Autodesk Fusion 360 part; units mm, degrees
(part 2 of 3)
  arc A151 (63.8462, -218.088) -> (64.9191, -217.0151) centre (64.9191, -218.088) cw
  line L279 (63.8462, -218.088) -> (63.8462, -226.6714)
  arc A152 (51.6032, -227.7443) -> (50.5303, -226.6714) centre (51.6032, -226.6714) cw
  line L280 (51.6032, -227.7443) -> (60.1866, -227.7443)
  arc A153 (61.2596, -226.6714) -> (60.1866, -227.7443) centre (60.1866, -226.6714) cw
  line L281 (61.2596, -226.6714) -> (61.2596, -218.088)
  arc A154 (60.1866, -217.0151) -> (61.2596, -218.088) centre (60.1866, -218.088) cw
  line L282 (60.1866, -217.0151) -> (51.6032, -217.0151)
  arc A155 (50.5303, -218.088) -> (51.6032, -217.0151) centre (51.6032, -218.088) cw
  line L283 (50.5303, -218.088) -> (50.5303, -226.6714)
  arc A156 (38.2293, -227.7443) -> (37.1563, -226.6714) centre (38.2293, -226.6714) cw
  line L284 (38.2293, -227.7443) -> (46.8127, -227.7443)
  arc A157 (47.8856, -226.6714) -> (46.8127, -227.7443) centre (46.8127, -226.6714) cw
  line L285 (47.8856, -226.6714) -> (47.8856, -218.088)
  arc A158 (46.8127, -217.0151) -> (47.8856, -218.088) centre (46.8127, -218.088) cw
  line L286 (46.8127, -217.0151) -> (38.2293, -217.0151)
  arc A159 (37.1563, -218.088) -> (38.2293, -217.0151) centre (38.2293, -218.088) cw
  line L287 (37.1563, -218.088) -> (37.1563, -226.6714)
  arc A160 (64.9191, -214.9497) -> (63.8462, -213.8768) centre (64.9191, -213.8768) cw
  line L288 (64.9191, -214.9497) -> (73.5025, -214.9497)
  arc A161 (74.5755, -213.8768) -> (73.5025, -214.9497) centre (73.5025, -213.8768) cw
  line L289 (74.5755, -213.8768) -> (74.5755, -205.2933)
  arc A162 (73.5025, -204.2204) -> (74.5755, -205.2933) centre (73.5025, -205.2934) cw
  line L290 (73.5025, -204.2204) -> (64.9191, -204.2204)
  arc A163 (63.8462, -205.2933) -> (64.9191, -204.2204) centre (64.9191, -205.2934) cw
  line L291 (63.8462, -205.2933) -> (63.8462, -213.8768)
  arc A164 (51.6032, -214.9497) -> (50.5303, -213.8768) centre (51.6032, -213.8768) cw
  line L292 (51.6032, -214.9497) -> (60.1866, -214.9497)
  arc A165 (61.2596, -213.8768) -> (60.1866, -214.9497) centre (60.1866, -213.8768) cw
  line L293 (61.2596, -213.8768) -> (61.2596, -205.2933)
  arc A166 (60.1866, -204.2204) -> (61.2596, -205.2933) centre (60.1866, -205.2934) cw
  line L294 (60.1866, -204.2204) -> (51.6032, -204.2204)
  arc A167 (50.5303, -205.2933) -> (51.6032, -204.2204) centre (51.6032, -205.2934) cw
  line L295 (50.5303, -205.2933) -> (50.5303, -213.8768)
  arc A168 (38.2293, -214.9497) -> (37.1563, -213.8768) centre (38.2293, -213.8768) cw
  line L296 (38.2293, -214.9497) -> (46.8127, -214.9497)
  arc A169 (47.8856, -213.8768) -> (46.8127, -214.9497) centre (46.8127, -213.8768) cw
  line L297 (47.8856, -213.8768) -> (47.8856, -205.2933)
  arc A170 (46.8127, -204.2204) -> (47.8856, -205.2933) centre (46.8127, -205.2934) cw
  line L298 (46.8127, -204.2204) -> (38.2293, -204.2204)
  arc A171 (37.1563, -205.2933) -> (38.2293, -204.2204) centre (38.2293, -205.2934) cw
  line L299 (37.1563, -205.2933) -> (37.1563, -213.8768)
  line L300 (53.9872, -39.8421) -> (53.9872, -39.7836)
  spline S12 degree 3 poles (53.9872, -39.7836) (53.9872, -38.4968) (55.0682, -37.4761) (56.4518, -37.4761) knots 0 0 0 0 1 1 1 1
  line L301 (56.4518, -37.4761) -> (133.5511, -37.4761)
  spline S13 degree 3 poles (133.5511, -37.4761) (134.8914, -37.4761) (136.0156, -38.5138) (136.0156, -39.8421) knots 0 0 0 0 1 1 1 1
  line L302 (136.0156, -39.8421) -> (136.0156, -39.9124)
  spline S14 degree 3 poles (136.0156, -39.9124) (136.0156, -41.1992) (134.9347, -42.2081) (133.5511, -42.2081) knots 0 0 0 0 1 1 1 1
  line L303 (133.5511, -42.2081) -> (56.4518, -42.2081)
  spline S15 degree 3 poles (56.4518, -42.2081) (55.1114, -42.2081) (53.9872, -41.1704) (53.9872, -39.8421) knots 0 0 0 0 1 1 1 1
  circle A172 centre (163.266, -40.5201) radius 1.3516
  circle A173 centre (26.8902, -40.575) radius 1.3516
  circle A174 centre (163.2802, -145.4039) radius 1.3516
  circle A175 centre (26.8546, -145.4321) radius 1.3516
  circle A176 centre (163.2436, -240.8365) radius 1.3516
  circle A177 centre (26.8198, -240.7999) radius 1.3516
  line L304 (146.1597, -138.0005) -> (151.9385, -138.0005)
  line L305 (152.9385, -139.0005) -> (152.9385, -146.7816)
  line L306 (151.9385, -147.7816) -> (146.1597, -147.7816)
  line L307 (145.1597, -146.7816) -> (145.1597, -139.0005)
  line L308 (146.1591, -150.9151) -> (151.9333, -150.9151)
  line L309 (152.9333, -151.9151) -> (152.9333, -159.6975)
  line L310 (151.9333, -160.6975) -> (146.1591, -160.6975)
  line L311 (145.1591, -159.6975) -> (145.1591, -151.9151)
  arc A178 (146.1597, -138.0005) -> (145.1597, -139.0005) centre (146.1597, -139.0005) ccw
  arc A179 (152.9385, -139.0005) -> (151.9385, -138.0005) centre (151.9385, -139.0005) ccw
  arc A180 (151.9385, -147.7816) -> (152.9385, -146.7816) centre (151.9385, -146.7816) ccw
  arc A181 (145.1597, -146.7816) -> (146.1597, -147.7816) centre (146.1597, -146.7816) ccw
  arc A182 (146.1591, -150.9151) -> (145.1591, -151.9151) centre (146.1591, -151.9151) ccw
  arc A183 (152.9333, -151.9151) -> (151.9333, -150.9151) centre (151.9333, -151.9151) ccw
  arc A184 (151.9333, -160.6975) -> (152.9333, -159.6975) centre (151.9333, -159.6975) ccw
  arc A185 (145.1591, -159.6975) -> (146.1591, -160.6975) centre (146.1591, -159.6975) ccw
  line L312 (22.9151, -34.1442) -> (167.1106, -34.1442)
  line L313 (168.1106, -35.1442) -> (168.1106, -260.4512)
  line L314 (167.1106, -261.4512) -> (22.9151, -261.4512)
  line L315 (21.9151, -260.4512) -> (21.9151, -35.1442)
  arc A186 (168.1106, -35.1442) -> (167.1106, -34.1442) centre (167.1106, -35.1442) ccw
  arc A187 (167.1106, -261.4512) -> (168.1106, -260.4512) centre (167.1106, -260.4512) ccw
  arc A188 (21.9151, -260.4512) -> (22.9151, -261.4512) centre (22.9151, -260.4512) ccw
  arc A189 (22.9151, -34.1442) -> (21.9151, -35.1442) centre (22.9151, -35.1442) ccw
  point P0 (164.6176, -40.5201)
  point P1 (28.2418, -40.575)
  point P2 (164.6318, -145.4039)
  point P3 (28.2062, -145.4321)
  point P4 (164.5952, -240.8365)
  point P5 (28.1714, -240.7999)
  dimension "d1" = 1
  dimension "d2" = 1
  constraint horizontal L304
  constraint vertical L305
  constraint horizontal L306
  constraint vertical L307
  constraint horizontal L308
  constraint vertical L309
  constraint horizontal L310
  constraint vertical L311
  constraint tangent L304 A178
  constraint tangent L307 A178
  constraint tangent L304 A179
  constraint tangent L305 A179
  constraint equal A178 A179
  constraint tangent L305 A180
  constraint tangent L306 A180
  constraint equal A178 A180
  constraint tangent L306 A181
  constraint tangent L307 A181
  constraint equal A178 A181
  constraint tangent L308 A182
  constraint tangent L311 A182
  constraint equal A178 A182
  constraint tangent L308 A183
  constraint tangent L309 A183
  constraint equal A178 A183
  constraint tangent L309 A184
  constraint tangent L310 A184
  constraint equal A178 A184
  constraint tangent L310 A185
  constraint tangent L311 A185
  constraint equal A178 A185
  constraint horizontal L312
  constraint vertical L313
  constraint horizontal L314
  constraint vertical L315
  constraint tangent L312 A186
  constraint tangent L313 A186
  constraint tangent L313 A187
  constraint tangent L314 A187
  constraint equal A186 A187
  constraint tangent L314 A188
  constraint tangent L315 A188
  constraint equal A186 A188
  constraint tangent L312 A189
  constraint tangent L315 A189
  constraint equal A186 A189
  measures "d1" radius of A178
  measures "d2" radius of A186
extrude "Extrude1" add sketch "Bottom" along normal blind 3
ref_plane "WorkPlane1" through (95.0128, -147.7977, 3) normal (0, 0, 1) x (1, 0, 0)
sketch "Middle" plane through (95.0128, -147.7977, 3) normal (0, 0, 1) x (1, 0, 0)
  arc A0 (-68.0338, 82.7631) -> (-69.035, 83.7643) centre (-68.0338, 83.7643) cw
  line L0 (-68.0338, 82.7631) -> (-59.5237, 82.7631)
  arc A1 (-58.5225, 83.7643) -> (-59.5237, 82.7631) centre (-59.5237, 83.7643) cw
  line L1 (-58.5225, 83.7643) -> (-58.5225, 88.4699)
  arc A2 (-59.5237, 89.4711) -> (-58.5225, 88.4699) centre (-59.5237, 88.4699) cw
  line L2 (-59.5237, 89.4711) -> (-68.0338, 89.4711)
  arc A3 (-69.035, 88.4699) -> (-68.0338, 89.4711) centre (-68.0338, 88.4699) cw
  line L3 (-69.035, 88.4699) -> (-69.035, 83.7643)
  arc A4 (-68.0338, 71.5687) -> (-69.035, 72.5699) centre (-68.0338, 72.5699) cw
  line L4 (-68.0338, 71.5687) -> (-59.5237, 71.5687)
  arc A5 (-58.5225, 72.5699) -> (-59.5237, 71.5687) centre (-59.5237, 72.5699) cw
  line L5 (-58.5225, 72.5699) -> (-58.5225, 77.2755)
  arc A6 (-59.5237, 78.2767) -> (-58.5225, 77.2755) centre (-59.5237, 77.2755) cw
  line L6 (-59.5237, 78.2767) -> (-68.0338, 78.2767)
  arc A7 (-69.035, 77.2755) -> (-68.0338, 78.2767) centre (-68.0338, 77.2755) cw
  line L7 (-69.035, 77.2755) -> (-69.035, 72.5699)
  arc A8 (-68.0338, 60.3295) -> (-69.035, 61.3307) centre (-68.0338, 61.3307) cw
  line L8 (-68.0338, 60.3295) -> (-59.5237, 60.3295)
  arc A9 (-58.5225, 61.3307) -> (-59.5237, 60.3295) centre (-59.5237, 61.3307) cw
  line L9 (-58.5225, 61.3307) -> (-58.5225, 66.0363)
  arc A10 (-59.5237, 67.0375) -> (-58.5225, 66.0363) centre (-59.5237, 66.0363) cw
  line L10 (-59.5237, 67.0375) -> (-68.0338, 67.0375)
  arc A11 (-69.035, 66.0363) -> (-68.0338, 67.0375) centre (-68.0338, 66.0363) cw
  line L11 (-69.035, 66.0363) -> (-69.035, 61.3307)
  arc A12 (-68.0338, 49.0663) -> (-69.035, 50.0675) centre (-68.0338, 50.0675) cw
  line L12 (-68.0338, 49.0663) -> (-59.5237, 49.0663)
  arc A13 (-58.5225, 50.0675) -> (-59.5237, 49.0663) centre (-59.5237, 50.0675) cw
  line L13 (-58.5225, 50.0675) -> (-58.5225, 54.7731)
  arc A14 (-59.5237, 55.7743) -> (-58.5225, 54.7731) centre (-59.5237, 54.7731) cw
  line L14 (-59.5237, 55.7743) -> (-68.0338, 55.7743)
  arc A15 (-69.035, 54.7731) -> (-68.0338, 55.7743) centre (-68.0338, 54.7731) cw
  line L15 (-69.035, 54.7731) -> (-69.035, 50.0675)
  arc A16 (-68.0338, 37.8539) -> (-69.035, 38.8551) centre (-68.0338, 38.8551) cw
  line L16 (-68.0338, 37.8539) -> (-59.5237, 37.8539)
  arc A17 (-58.5225, 38.8551) -> (-59.5237, 37.8539) centre (-59.5237, 38.8551) cw
  line L17 (-58.5225, 38.8551) -> (-58.5225, 43.5607)
  arc A18 (-59.5237, 44.5619) -> (-58.5225, 43.5607) centre (-59.5237, 43.5607) cw
  line L18 (-59.5237, 44.5619) -> (-68.0338, 44.5619)
  arc A19 (-69.035, 43.5607) -> (-68.0338, 44.5619) centre (-68.0338, 43.5607) cw
  line L19 (-69.035, 43.5607) -> (-69.035, 38.8551)
  arc A20 (-68.0338, 26.6171) -> (-69.035, 27.6183) centre (-68.0338, 27.6183) cw
  line L20 (-68.0338, 26.6171) -> (-59.5237, 26.6171)
  arc A21 (-58.5225, 27.6183) -> (-59.5237, 26.6171) centre (-59.5237, 27.6183) cw
  line L21 (-58.5225, 27.6183) -> (-58.5225, 32.3239)
  arc A22 (-59.5237, 33.3251) -> (-58.5225, 32.3239) centre (-59.5237, 32.3239) cw
  line L22 (-59.5237, 33.3251) -> (-68.0338, 33.3251)
  arc A23 (-69.035, 32.3239) -> (-68.0338, 33.3251) centre (-68.0338, 32.3239) cw
  line L23 (-69.035, 32.3239) -> (-69.035, 27.6183)
  arc A24 (59.9614, 26.5376) -> (58.9602, 27.5388) centre (59.9614, 27.5388) cw
  line L24 (59.9614, 26.5376) -> (68.4716, 26.5376)
  arc A25 (69.4728, 27.5388) -> (68.4716, 26.5376) centre (68.4716, 27.5388) cw
  line L25 (69.4728, 27.5388) -> (69.4728, 32.2444)
  arc A26 (68.4716, 33.2456) -> (69.4728, 32.2444) centre (68.4716, 32.2444) cw
  line L26 (68.4716, 33.2456) -> (59.9614, 33.2456)
  arc A27 (58.9602, 32.2444) -> (59.9614, 33.2456) centre (59.9614, 32.2444) cw
  line L27 (58.9602, 32.2444) -> (58.9602, 27.5388)
  arc A28 (59.9614, 37.7744) -> (58.9602, 38.7756) centre (59.9614, 38.7756) cw
  line L28 (59.9614, 37.7744) -> (68.4716, 37.7744)
  arc A29 (69.4728, 38.7756) -> (68.4716, 37.7744) centre (68.4716, 38.7756) cw
  line L29 (69.4728, 38.7756) -> (69.4728, 43.4812)
  arc A30 (68.4716, 44.4824) -> (69.4728, 43.4812) centre (68.4716, 43.4812) cw
  line L30 (68.4716, 44.4824) -> (59.9614, 44.4824)
  arc A31 (58.9602, 43.4812) -> (59.9614, 44.4824) centre (59.9614, 43.4812) cw
  line L31 (58.9602, 43.4812) -> (58.9602, 38.7756)
  arc A32 (59.9614, 49.0133) -> (58.9602, 50.0145) centre (59.9614, 50.0145) cw
  line L32 (59.9614, 49.0133) -> (68.4716, 49.0133)
  arc A33 (69.4728, 50.0145) -> (68.4716, 49.0133) centre (68.4716, 50.0145) cw
  line L33 (69.4728, 50.0145) -> (69.4728, 54.7201)
  arc A34 (68.4716, 55.7213) -> (69.4728, 54.7201) centre (68.4716, 54.7201) cw
  line L34 (68.4716, 55.7213) -> (59.9614, 55.7213)
  arc A35 (58.9602, 54.7201) -> (59.9614, 55.7213) centre (59.9614, 54.7201) cw
  line L35 (58.9602, 54.7201) -> (58.9602, 50.0145)
  arc A36 (59.9614, 60.2236) -> (58.9602, 61.2248) centre (59.9614, 61.2248) cw
  line L36 (59.9614, 60.2236) -> (68.4716, 60.2236)
  arc A37 (69.4728, 61.2248) -> (68.4716, 60.2236) centre (68.4716, 61.2248) cw
  line L37 (69.4728, 61.2248) -> (69.4728, 65.9304)
  arc A38 (68.4716, 66.9316) -> (69.4728, 65.9304) centre (68.4716, 65.9304) cw
  line L38 (68.4716, 66.9316) -> (59.9614, 66.9316)
  arc A39 (58.9602, 65.9304) -> (59.9614, 66.9316) centre (59.9614, 65.9304) cw
  line L39 (58.9602, 65.9304) -> (58.9602, 61.2248)
  arc A40 (59.9614, 71.4892) -> (58.9602, 72.4904) centre (59.9614, 72.4904) cw
  line L40 (59.9614, 71.4892) -> (68.4716, 71.4892)
  arc A41 (69.4728, 72.4904) -> (68.4716, 71.4892) centre (68.4716, 72.4904) cw
  line L41 (69.4728, 72.4904) -> (69.4728, 77.196)
  arc A42 (68.4716, 78.1972) -> (69.4728, 77.196) centre (68.4716, 77.196) cw
  line L42 (68.4716, 78.1972) -> (59.9614, 78.1972)
  arc A43 (58.9602, 77.196) -> (59.9614, 78.1972) centre (59.9614, 77.196) cw
  line L43 (58.9602, 77.196) -> (58.9602, 72.4904)
  arc A44 (59.9614, 82.7631) -> (58.9602, 83.7643) centre (59.9614, 83.7643) cw
  line L44 (59.9614, 82.7631) -> (68.4716, 82.7631)
  arc A45 (69.4728, 83.7643) -> (68.4716, 82.7631) centre (68.4716, 83.7643) cw
  line L45 (69.4728, 83.7643) -> (69.4728, 88.4699)
  arc A46 (68.4716, 89.4711) -> (69.4728, 88.4699) centre (68.4716, 88.4699) cw
  line L46 (68.4716, 89.4711) -> (59.9614, 89.4711)
  arc A47 (58.9602, 88.4699) -> (59.9614, 89.4711) centre (59.9614, 88.4699) cw
  line L47 (58.9602, 88.4699) -> (58.9602, 83.7643)
  arc A48 (-54.8782, 0.767) -> (-55.8794, 1.7682) centre (-54.8782, 1.7682) cw
  line L48 (-54.8782, 0.767) -> (-43.6448, 0.767)
  arc A49 (-42.6436, 1.7682) -> (-43.6448, 0.767) centre (-43.6448, 1.7682) cw
  line L49 (-42.6436, 1.7682) -> (-42.6436, 7.8755)
  arc A50 (-43.6448, 8.8767) -> (-42.6436, 7.8755) centre (-43.6448, 7.8755) cw
  line L50 (-43.6448, 8.8767) -> (-54.8782, 8.8767)
  arc A51 (-55.8794, 7.8755) -> (-54.8782, 8.8767) centre (-54.8782, 7.8755) cw
  line L51 (-55.8794, 7.8755) -> (-55.8794, 1.7682)
  arc A52 (-54.8782, -12.0499) -> (-55.8794, -11.0487) centre (-54.8782, -11.0487) cw
  line L52 (-54.8782, -12.0499) -> (-43.6448, -12.0499)
  arc A53 (-42.6436, -11.0487) -> (-43.6448, -12.0499) centre (-43.6448, -11.0487) cw
  line L53 (-42.6436, -11.0487) -> (-42.6436, -4.9414)
  arc A54 (-43.6448, -3.9402) -> (-42.6436, -4.9414) centre (-43.6448, -4.9414) cw
  line L54 (-43.6448, -3.9402) -> (-54.8782, -3.9402)
  arc A55 (-55.8794, -4.9414) -> (-54.8782, -3.9402) centre (-54.8782, -4.9414) cw
  line L55 (-55.8794, -4.9414) -> (-55.8794, -11.0487)
  arc A56 (-54.8782, -25.4495) -> (-55.8794, -24.4483) centre (-54.8782, -24.4483) cw
  line L56 (-54.8782, -25.4495) -> (-43.6448, -25.4495)
  arc A57 (-42.6436, -24.4483) -> (-43.6448, -25.4495) centre (-43.6448, -24.4483) cw
  line L57 (-42.6436, -24.4483) -> (-42.6436, -18.3411)
  arc A58 (-43.6448, -17.3399) -> (-42.6436, -18.3411) centre (-43.6448, -18.3411) cw
  line L58 (-43.6448, -17.3399) -> (-54.8782, -17.3399)
  arc A59 (-55.8794, -18.3411) -> (-54.8782, -17.3399) centre (-54.8782, -18.3411) cw
  line L59 (-55.8794, -18.3411) -> (-55.8794, -24.4483)
  arc A60 (-54.8782, -38.5373) -> (-55.8794, -37.5362) centre (-54.8782, -37.5362) cw
  line L60 (-54.8782, -38.5373) -> (-43.6448, -38.5373)
  arc A61 (-42.6436, -37.5362) -> (-43.6448, -38.5373) centre (-43.6448, -37.5362) cw
  line L61 (-42.6436, -37.5362) -> (-42.6436, -31.4289)
  arc A62 (-43.6448, -30.4277) -> (-42.6436, -31.4289) centre (-43.6448, -31.4289) cw
  line L62 (-43.6448, -30.4277) -> (-54.8782, -30.4277)
  arc A63 (-55.8794, -31.4289) -> (-54.8782, -30.4277) centre (-54.8782, -31.4289) cw
  line L63 (-55.8794, -31.4289) -> (-55.8794, -37.5362)
  arc A64 (-54.8782, -51.5721) -> (-55.8794, -50.5709) centre (-54.8782, -50.5709) cw
  line L64 (-54.8782, -51.5721) -> (-43.6448, -51.5721)
  arc A65 (-42.6436, -50.5709) -> (-43.6448, -51.5721) centre (-43.6448, -50.5709) cw
  line L65 (-42.6436, -50.5709) -> (-42.6436, -44.4636)
  arc A66 (-43.6448, -43.4624) -> (-42.6436, -44.4636) centre (-43.6448, -44.4636) cw
  line L66 (-43.6448, -43.4624) -> (-54.8782, -43.4624)
  arc A67 (-55.8794, -44.4636) -> (-54.8782, -43.4624) centre (-54.8782, -44.4636) cw
  line L67 (-55.8794, -44.4636) -> (-55.8794, -50.5709)
  arc A68 (-36.9816, -51.5721) -> (-37.9828, -50.5709) centre (-36.9816, -50.5709) cw
  line L68 (-36.9816, -51.5721) -> (-25.7482, -51.5721)
  arc A69 (-24.747, -50.5709) -> (-25.7482, -51.5721) centre (-25.7482, -50.5709) cw
  line L69 (-24.747, -50.5709) -> (-24.747, -44.4636)
  arc A70 (-25.7482, -43.4624) -> (-24.747, -44.4636) centre (-25.7482, -44.4636) cw
  line L70 (-25.7482, -43.4624) -> (-36.9816, -43.4624)
  arc A71 (-37.9828, -44.4636) -> (-36.9816, -43.4624) centre (-36.9816, -44.4636) cw
  line L71 (-37.9828, -44.4636) -> (-37.9828, -50.5709)
  arc A72 (-36.9816, -38.5373) -> (-37.9828, -37.5362) centre (-36.9816, -37.5362) cw
  line L72 (-36.9816, -38.5373) -> (-25.7482, -38.5373)
  arc A73 (-24.747, -37.5362) -> (-25.7482, -38.5373) centre (-25.7482, -37.5362) cw
  line L73 (-24.747, -37.5362) -> (-24.747, -31.4289)
  arc A74 (-25.7482, -30.4277) -> (-24.747, -31.4289) centre (-25.7482, -31.4289) cw
  line L74 (-25.7482, -30.4277) -> (-36.9816, -30.4277)
  arc A75 (-37.9828, -31.4289) -> (-36.9816, -30.4277) centre (-36.9816, -31.4289) cw
  line L75 (-37.9828, -31.4289) -> (-37.9828, -37.5362)
  arc A76 (-36.9816, -25.4495) -> (-37.9828, -24.4483) centre (-36.9816, -24.4483) cw
  line L76 (-36.9816, -25.4495) -> (-25.7482, -25.4495)
  arc A77 (-24.747, -24.4483) -> (-25.7482, -25.4495) centre (-25.7482, -24.4483) cw
  line L77 (-24.747, -24.4483) -> (-24.747, -18.3411)
  arc A78 (-25.7482, -17.3399) -> (-24.747, -18.3411) centre (-25.7482, -18.3411) cw
  line L78 (-25.7482, -17.3399) -> (-36.9816, -17.3399)
  arc A79 (-37.9828, -18.3411) -> (-36.9816, -17.3399) centre (-36.9816, -18.3411) cw
  line L79 (-37.9828, -18.3411) -> (-37.9828, -24.4483)
  arc A80 (-36.9816, -12.0499) -> (-37.9828, -11.0487) centre (-36.9816, -11.0487) cw
  line L80 (-36.9816, -12.0499) -> (-25.7482, -12.0499)
  arc A81 (-24.747, -11.0487) -> (-25.7482, -12.0499) centre (-25.7482, -11.0487) cw
  line L81 (-24.747, -11.0487) -> (-24.747, -4.9414)
  arc A82 (-25.7482, -3.9402) -> (-24.747, -4.9414) centre (-25.7482, -4.9414) cw
  line L82 (-25.7482, -3.9402) -> (-36.9816, -3.9402)
  arc A83 (-37.9828, -4.9414) -> (-36.9816, -3.9402) centre (-36.9816, -4.9414) cw
  line L83 (-37.9828, -4.9414) -> (-37.9828, -11.0487)
  arc A84 (-36.9816, 0.767) -> (-37.9828, 1.7682) centre (-36.9816, 1.7682) cw
  line L84 (-36.9816, 0.767) -> (-25.7482, 0.767)
  arc A85 (-24.747, 1.7682) -> (-25.7482, 0.767) centre (-25.7482, 1.7682) cw
  line L85 (-24.747, 1.7682) -> (-24.747, 7.8755)
  arc A86 (-25.7482, 8.8767) -> (-24.747, 7.8755) centre (-25.7482, 7.8755) cw
  line L86 (-25.7482, 8.8767) -> (-36.9816, 8.8767)
  arc A87 (-37.9828, 7.8755) -> (-36.9816, 8.8767) centre (-36.9816, 7.8755) cw
  line L87 (-37.9828, 7.8755) -> (-37.9828, 1.7682)
  arc A88 (-18.8211, 0.767) -> (-19.8223, 1.7682) centre (-18.8211, 1.7682) cw
  line L88 (-18.8211, 0.767) -> (-7.5877, 0.767)
  arc A89 (-6.5865, 1.7682) -> (-7.5877, 0.767) centre (-7.5877, 1.7682) cw
  line L89 (-6.5865, 1.7682) -> (-6.5865, 7.8755)
  arc A90 (-7.5877, 8.8767) -> (-6.5865, 7.8755) centre (-7.5877, 7.8755) cw
  line L90 (-7.5877, 8.8767) -> (-18.8211, 8.8767)
  arc A91 (-19.8223, 7.8755) -> (-18.8211, 8.8767) centre (-18.8211, 7.8755) cw
  line L91 (-19.8223, 7.8755) -> (-19.8223, 1.7682)
  arc A92 (-18.8211, -12.0499) -> (-19.8223, -11.0487) centre (-18.8211, -11.0487) cw
  line L92 (-18.8211, -12.0499) -> (-7.5877, -12.0499)
  arc A93 (-6.5865, -11.0487) -> (-7.5877, -12.0499) centre (-7.5877, -11.0487) cw
  line L93 (-6.5865, -11.0487) -> (-6.5865, -4.9414)
  arc A94 (-7.5877, -3.9402) -> (-6.5865, -4.9414) centre (-7.5877, -4.9414) cw
  line L94 (-7.5877, -3.9402) -> (-18.8211, -3.9402)
  arc A95 (-19.8223, -4.9414) -> (-18.8211, -3.9402) centre (-18.8211, -4.9414) cw
  line L95 (-19.8223, -4.9414) -> (-19.8223, -11.0487)
  arc A96 (-0.6342, 0.767) -> (-1.6354, 1.7682) centre (-0.6342, 1.7682) cw
  line L96 (-0.6342, 0.767) -> (10.5992, 0.767)
  arc A97 (11.6004, 1.7682) -> (10.5992, 0.767) centre (10.5992, 1.7682) cw
  line L97 (11.6004, 1.7682) -> (11.6004, 7.8755)
  arc A98 (10.5992, 8.8767) -> (11.6004, 7.8755) centre (10.5992, 7.8755) cw
  line L98 (10.5992, 8.8767) -> (-0.6342, 8.8767)
  arc A99 (-1.6354, 7.8755) -> (-0.6342, 8.8767) centre (-0.6342, 7.8755) cw
  line L99 (-1.6354, 7.8755) -> (-1.6354, 1.7682)
  arc A100 (-0.6342, -12.0499) -> (-1.6354, -11.0487) centre (-0.6342, -11.0487) cw
  line L100 (-0.6342, -12.0499) -> (10.5992, -12.0499)
  arc A101 (11.6004, -11.0487) -> (10.5992, -12.0499) centre (10.5992, -11.0487) cw
  line L101 (11.6004, -11.0487) -> (11.6004, -4.9414)
  arc A102 (10.5992, -3.9402) -> (11.6004, -4.9414) centre (10.5992, -4.9414) cw
  line L102 (10.5992, -3.9402) -> (-0.6342, -3.9402)
  arc A103 (-1.6354, -4.9414) -> (-0.6342, -3.9402) centre (-0.6342, -4.9414) cw
  line L103 (-1.6354, -4.9414) -> (-1.6354, -11.0487)
  arc A104 (17.3673, 0.767) -> (16.3662, 1.7682) centre (17.3673, 1.7682) cw
  line L104 (17.3673, 0.767) -> (28.6008, 0.767)
  arc A105 (29.602, 1.7682) -> (28.6008, 0.767) centre (28.6008, 1.7682) cw
  line L105 (29.602, 1.7682) -> (29.602, 7.8755)
  arc A106 (28.6008, 8.8767) -> (29.602, 7.8755) centre (28.6008, 7.8755) cw
  line L106 (28.6008, 8.8767) -> (17.3673, 8.8767)
  arc A107 (16.3662, 7.8755) -> (17.3673, 8.8767) centre (17.3673, 7.8755) cw
  line L107 (16.3662, 7.8755) -> (16.3662, 1.7682)
  arc A108 (17.3673, -12.0499) -> (16.3662, -11.0487) centre (17.3673, -11.0487) cw
  line L108 (17.3673, -12.0499) -> (28.6008, -12.0499)
  arc A109 (29.602, -11.0487) -> (28.6008, -12.0499) centre (28.6008, -11.0487) cw
  line L109 (29.602, -11.0487) -> (29.602, -4.9414)
  arc A110 (28.6008, -3.9402) -> (29.602, -4.9414) centre (28.6008, -4.9414) cw
  line L110 (28.6008, -3.9402) -> (17.3673, -3.9402)
  arc A111 (16.3662, -4.9414) -> (17.3673, -3.9402) centre (17.3673, -4.9414) cw
  line L111 (16.3662, -4.9414) -> (16.3662, -11.0487)
  arc A112 (35.4483, 0.767) -> (34.4471, 1.7682) centre (35.4483, 1.7682) cw
  line L112 (35.4483, 0.767) -> (46.6818, 0.767)
  arc A113 (47.6829, 1.7682) -> (46.6818, 0.767) centre (46.6817, 1.7682) cw
  line L113 (47.6829, 1.7682) -> (47.6829, 7.8755)
  arc A114 (46.6817, 8.8767) -> (47.6829, 7.8755) centre (46.6817, 7.8755) cw
  line L114 (46.6817, 8.8767) -> (35.4483, 8.8767)
  arc A115 (34.4471, 7.8755) -> (35.4483, 8.8767) centre (35.4483, 7.8755) cw
  line L115 (34.4471, 7.8755) -> (34.4471, 1.7682)
  arc A116 (35.4483, -12.0499) -> (34.4471, -11.0487) centre (35.4483, -11.0487) cw
  line L116 (35.4483, -12.0499) -> (46.6818, -12.0499)
  arc A117 (47.6829, -11.0487) -> (46.6818, -12.0499) centre (46.6817, -11.0487) cw
  line L117 (47.6829, -11.0487) -> (47.6829, -4.9414)
  arc A118 (46.6817, -3.9402) -> (47.6829, -4.9414) centre (46.6817, -4.9414) cw
  line L118 (46.6817, -3.9402) -> (35.4483, -3.9402)
  arc A119 (34.4471, -4.9414) -> (35.4483, -3.9402) centre (35.4483, -4.9414) cw
  line L119 (34.4471, -4.9414) -> (34.4471, -11.0487)
  arc A120 (31.3954, -29.6551) -> (30.3942, -28.6539) centre (31.3954, -28.6539) cw
  line L120 (31.3954, -29.6551) -> (39.405, -29.6551)
  arc A121 (40.4061, -28.6539) -> (39.405, -29.6551) centre (39.405, -28.6539) cw
  line L121 (40.4061, -28.6539) -> (40.4061, -20.6443)
  arc A122 (39.405, -19.6431) -> (40.4061, -20.6443) centre (39.405, -20.6443) cw
  line L122 (39.405, -19.6431) -> (31.3954, -19.6431)
  arc A123 (30.3942, -20.6443) -> (31.3954, -19.6431) centre (31.3954, -20.6443) cw
  line L123 (30.3942, -20.6443) -> (30.3942, -28.6539)
  arc A124 (46.3835, -29.614) -> (45.3823, -28.6128) centre (46.3835, -28.6128) cw
  line L124 (46.3835, -29.614) -> (54.3931, -29.614)
  arc A125 (55.3943, -28.6128) -> (54.3931, -29.614) centre (54.3931, -28.6128) cw
  line L125 (55.3943, -28.6128) -> (55.3943, -20.6033)
  arc A126 (54.3931, -19.6021) -> (55.3943, -20.6033) centre (54.3931, -20.6033) cw
  line L126 (54.3931, -19.6021) -> (46.3835, -19.6021)
  arc A127 (45.3823, -20.6033) -> (46.3835, -19.6021) centre (46.3835, -20.6033) cw
  line L127 (45.3823, -20.6033) -> (45.3823, -28.6128)
  arc A128 (-13.9242, -29.6551) -> (-14.9253, -28.6539) centre (-13.9242, -28.6539) cw
  line L128 (-13.9242, -29.6551) -> (-5.9146, -29.6551)
  arc A129 (-4.9134, -28.6539) -> (-5.9146, -29.6551) centre (-5.9146, -28.6539) cw
  line L129 (-4.9134, -28.6539) -> (-4.9134, -20.6443)
  arc A130 (-5.9146, -19.6431) -> (-4.9134, -20.6443) centre (-5.9146, -20.6443) cw
  line L130 (-5.9146, -19.6431) -> (-13.9242, -19.6431)
  arc A131 (-14.9253, -20.6443) -> (-13.9242, -19.6431) centre (-13.9242, -20.6443) cw
  line L131 (-14.9253, -20.6443) -> (-14.9253, -28.6539)
  arc A132 (1.1007, -29.6551) -> (0.0995, -28.6539) centre (1.1007, -28.6539) cw
  line L132 (1.1007, -29.6551) -> (9.1102, -29.6551)
  arc A133 (10.1114, -28.6539) -> (9.1102, -29.6551) centre (9.1102, -28.6539) cw
  line L133 (10.1114, -28.6539) -> (10.1114, -20.6443)
  arc A134 (9.1103, -19.6431) -> (10.1114, -20.6443) centre (9.1102, -20.6443) cw
  line L134 (9.1103, -19.6431) -> (1.1007, -19.6431)
  arc A135 (0.0995, -20.6443) -> (1.1007, -19.6431) centre (1.1007, -20.6443) cw
  line L135 (0.0995, -20.6443) -> (0.0995, -28.6539)
  arc A136 (16.2654, -29.6551) -> (15.2642, -28.6539) centre (16.2654, -28.6539) cw
  line L136 (16.2654, -29.6551) -> (24.275, -29.6551)
  arc A137 (25.2761, -28.6539) -> (24.275, -29.6551) centre (24.275, -28.6539) cw
  line L137 (25.2761, -28.6539) -> (25.2761, -20.6443)
  arc A138 (24.275, -19.6431) -> (25.2761, -20.6443) centre (24.275, -20.6443) cw
  line L138 (24.275, -19.6431) -> (16.2654, -19.6431)
  arc A139 (15.2642, -20.6443) -> (16.2654, -19.6431) centre (16.2654, -20.6443) cw
  line L139 (15.2642, -20.6443) -> (15.2642, -28.6539)
  arc A140 (46.3835, -44.5902) -> (45.3823, -43.589) centre (46.3835, -43.589) cw
  line L140 (46.3835, -44.5902) -> (54.3931, -44.5902)
  arc A141 (55.3943, -43.589) -> (54.3931, -44.5902) centre (54.3931, -43.589) cw
  line L141 (55.3943, -43.589) -> (55.3943, -35.5795)
  arc A142 (54.3931, -34.5783) -> (55.3943, -35.5795) centre (54.3931, -35.5795) cw
  line L142 (54.3931, -34.5783) -> (46.3835, -34.5783)
  arc A143 (45.3823, -35.5795) -> (46.3835, -34.5783) centre (46.3835, -35.5795) cw
  line L143 (45.3823, -35.5795) -> (45.3823, -43.589)
  arc A144 (31.3954, -44.6313) -> (30.3942, -43.6301) centre (31.3954, -43.6301) cw
  line L144 (31.3954, -44.6313) -> (39.405, -44.6313)
  arc A145 (40.4061, -43.6301) -> (39.405, -44.6313) centre (39.405, -43.6301) cw
  line L145 (40.4061, -43.6301) -> (40.4061, -35.6205)
  arc A146 (39.405, -34.6193) -> (40.4061, -35.6205) centre (39.405, -35.6205) cw
  line L146 (39.405, -34.6193) -> (31.3954, -34.6193)
  arc A147 (30.3942, -35.6205) -> (31.3954, -34.6193) centre (31.3954, -35.6205) cw
  line L147 (30.3942, -35.6205) -> (30.3942, -43.6301)
  arc A148 (16.2654, -44.6313) -> (15.2642, -43.6301) centre (16.2654, -43.6301) cw
  line L148 (16.2654, -44.6313) -> (24.275, -44.6313)
  arc A149 (25.2761, -43.6301) -> (24.275, -44.6313) centre (24.275, -43.6301) cw
  line L149 (25.2761, -43.6301) -> (25.2761, -35.6205)
  arc A150 (24.275, -34.6193) -> (25.2761, -35.6205) centre (24.275, -35.6205) cw
  line L150 (24.275, -34.6193) -> (16.2654, -34.6193)
  arc A151 (15.2642, -35.6205) -> (16.2654, -34.6193) centre (16.2654, -35.6205) cw
  line L151 (15.2642, -35.6205) -> (15.2642, -43.6301)
  arc A152 (1.1007, -44.6313) -> (0.0995, -43.6301) centre (1.1007, -43.6301) cw
  line L152 (1.1007, -44.6313) -> (9.1102, -44.6313)
  arc A153 (10.1114, -43.6301) -> (9.1102, -44.6313) centre (9.1102, -43.6301) cw
  line L153 (10.1114, -43.6301) -> (10.1114, -35.6205)
  arc A154 (9.1103, -34.6193) -> (10.1114, -35.6205) centre (9.1102, -35.6205) cw
  line L154 (9.1103, -34.6193) -> (1.1007, -34.6193)
  arc A155 (0.0995, -35.6205) -> (1.1007, -34.6193) centre (1.1007, -35.6205) cw
  line L155 (0.0995, -35.6205) -> (0.0995, -43.6301)
  arc A156 (-13.9242, -44.6313) -> (-14.9253, -43.6301) centre (-13.9242, -43.6301) cw
  line L156 (-13.9242, -44.6313) -> (-5.9146, -44.6313)
  arc A157 (-4.9134, -43.6301) -> (-5.9146, -44.6313) centre (-5.9146, -43.6301) cw
  line L157 (-4.9134, -43.6301) -> (-4.9134, -35.6205)
  arc A158 (-5.9146, -34.6193) -> (-4.9134, -35.6205) centre (-5.9146, -35.6205) cw
  line L158 (-5.9146, -34.6193) -> (-13.9242, -34.6193)
  arc A159 (-14.9253, -35.6205) -> (-13.9242, -34.6193) centre (-13.9242, -35.6205) cw
  line L159 (-14.9253, -35.6205) -> (-14.9253, -43.6301)
  arc A160 (46.3835, -59.646) -> (45.3823, -58.6448) centre (46.3835, -58.6448) cw
  line L160 (46.3835, -59.646) -> (54.3931, -59.646)
  arc A161 (55.3943, -58.6448) -> (54.3931, -59.646) centre (54.3931, -58.6448) cw
  line L161 (55.3943, -58.6448) -> (55.3943, -50.6352)
  arc A162 (54.3931, -49.634) -> (55.3943, -50.6352) centre (54.3931, -50.6352) cw
  line L162 (54.3931, -49.634) -> (46.3835, -49.634)
  arc A163 (45.3823, -50.6352) -> (46.3835, -49.634) centre (46.3835, -50.6352) cw
  line L163 (45.3823, -50.6352) -> (45.3823, -58.6448)
  arc A164 (31.3954, -59.687) -> (30.3942, -58.6858) centre (31.3954, -58.6858) cw
  line L164 (31.3954, -59.687) -> (39.405, -59.687)
  arc A165 (40.4061, -58.6858) -> (39.405, -59.687) centre (39.405, -58.6858) cw
  line L165 (40.4061, -58.6858) -> (40.4061, -50.6763)
  arc A166 (39.405, -49.6751) -> (40.4061, -50.6763) centre (39.405, -50.6763) cw
  line L166 (39.405, -49.6751) -> (31.3954, -49.6751)
  arc A167 (30.3942, -50.6763) -> (31.3954, -49.6751) centre (31.3954, -50.6763) cw
  line L167 (30.3942, -50.6763) -> (30.3942, -58.6858)
  arc A168 (16.2654, -59.687) -> (15.2642, -58.6858) centre (16.2654, -58.6858) cw
  line L168 (16.2654, -59.687) -> (24.275, -59.687)
  arc A169 (25.2761, -58.6858) -> (24.275, -59.687) centre (24.275, -58.6858) cw
  line L169 (25.2761, -58.6858) -> (25.2761, -50.6763)
  arc A170 (24.275, -49.6751) -> (25.2761, -50.6763) centre (24.275, -50.6763) cw
  line L170 (24.275, -49.6751) -> (16.2654, -49.6751)
  arc A171 (15.2642, -50.6763) -> (16.2654, -49.6751) centre (16.2654, -50.6763) cw
  line L171 (15.2642, -50.6763) -> (15.2642, -58.6858)
  arc A172 (1.1007, -59.687) -> (0.0995, -58.6858) centre (1.1007, -58.6858) cw
  line L172 (1.1007, -59.687) -> (9.1102, -59.687)
  arc A173 (10.1114, -58.6858) -> (9.1102, -59.687) centre (9.1102, -58.6858) cw
  line L173 (10.1114, -58.6858) -> (10.1114, -50.6763)
  arc A174 (9.1103, -49.6751) -> (10.1114, -50.6763) centre (9.1102, -50.6763) cw
  line L174 (9.1103, -49.6751) -> (1.1007, -49.6751)
  arc A175 (0.0995, -50.6763) -> (1.1007, -49.6751) centre (1.1007, -50.6763) cw
  line L175 (0.0995, -50.6763) -> (0.0995, -58.6858)
  arc A176 (-13.9242, -59.687) -> (-14.9253, -58.6858) centre (-13.9242, -58.6858) cw
  line L176 (-13.9242, -59.687) -> (-5.9146, -59.687)
  arc A177 (-4.9134, -58.6858) -> (-5.9146, -59.687) centre (-5.9146, -58.6858) cw
  line L177 (-4.9134, -58.6858) -> (-4.9134, -50.6763)
  arc A178 (-5.9146, -49.6751) -> (-4.9134, -50.6763) centre (-5.9146, -50.6763) cw
  line L178 (-5.9146, -49.6751) -> (-13.9242, -49.6751)
  arc A179 (-14.9253, -50.6763) -> (-13.9242, -49.6751) centre (-13.9242, -50.6763) cw
  line L179 (-14.9253, -50.6763) -> (-14.9253, -58.6858)
  arc A180 (46.3835, -74.675) -> (45.3823, -73.6738) centre (46.3835, -73.6738) cw
  line L180 (46.3835, -74.675) -> (54.3931, -74.675)
  arc A181 (55.3943, -73.6738) -> (54.3931, -74.675) centre (54.3931, -73.6738) cw
  line L181 (55.3943, -73.6738) -> (55.3943, -65.6643)
  arc A182 (54.3931, -64.6631) -> (55.3943, -65.6643) centre (54.3931, -65.6643) cw
  line L182 (54.3931, -64.6631) -> (46.3835, -64.6631)
  arc A183 (45.3823, -65.6643) -> (46.3835, -64.6631) centre (46.3835, -65.6643) cw
  line L183 (45.3823, -65.6643) -> (45.3823, -73.6738)
  arc A184 (31.3954, -74.7161) -> (30.3942, -73.7149) centre (31.3954, -73.7149) cw
  line L184 (31.3954, -74.7161) -> (39.405, -74.7161)
  arc A185 (40.4061, -73.7149) -> (39.405, -74.7161) centre (39.405, -73.7149) cw
  line L185 (40.4061, -73.7149) -> (40.4061, -65.7053)
  arc A186 (39.405, -64.7041) -> (40.4061, -65.7053) centre (39.405, -65.7053) cw
  line L186 (39.405, -64.7041) -> (31.3954, -64.7041)
  arc A187 (30.3942, -65.7054) -> (31.3954, -64.7041) centre (31.3954, -65.7053) cw
  line L187 (30.3942, -65.7054) -> (30.3942, -73.7149)
  arc A188 (16.2654, -74.7161) -> (15.2642, -73.7149) centre (16.2654, -73.7149) cw
  line L188 (16.2654, -74.7161) -> (24.275, -74.7161)
  arc A189 (25.2761, -73.7149) -> (24.275, -74.7161) centre (24.275, -73.7149) cw
  line L189 (25.2761, -73.7149) -> (25.2761, -65.7053)
  arc A190 (24.275, -64.7041) -> (25.2761, -65.7053) centre (24.275, -65.7053) cw
  line L190 (24.275, -64.7041) -> (16.2654, -64.7041)
  arc A191 (15.2642, -65.7054) -> (16.2654, -64.7041) centre (16.2654, -65.7053) cw
  line L191 (15.2642, -65.7054) -> (15.2642, -73.7149)
  arc A192 (1.1007, -74.7161) -> (0.0995, -73.7149) centre (1.1007, -73.7149) cw
  line L192 (1.1007, -74.7161) -> (9.1102, -74.7161)
  arc A193 (10.1114, -73.7149) -> (9.1102, -74.7161) centre (9.1102, -73.7149) cw
  line L193 (10.1114, -73.7149) -> (10.1114, -65.7053)
  arc A194 (9.1103, -64.7041) -> (10.1114, -65.7053) centre (9.1102, -65.7053) cw
  line L194 (9.1103, -64.7041) -> (1.1007, -64.7041)
  arc A195 (0.0995, -65.7054) -> (1.1007, -64.7041) centre (1.1007, -65.7053) cw
  line L195 (0.0995, -65.7054) -> (0.0995, -73.7149)
  arc A196 (-13.9242, -74.7161) -> (-14.9253, -73.7149) centre (-13.9242, -73.7149) cw
  line L196 (-13.9242, -74.7161) -> (-5.9146, -74.7161)
  arc A197 (-4.9134, -73.7149) -> (-5.9146, -74.7161) centre (-5.9146, -73.7149) cw
  line L197 (-4.9134, -73.7149) -> (-4.9134, -65.7053)
  arc A198 (-5.9146, -64.7041) -> (-4.9134, -65.7053) centre (-5.9146, -65.7053) cw
  line L198 (-5.9146, -64.7041) -> (-13.9242, -64.7041)
  arc A199 (-14.9253, -65.7054) -> (-13.9242, -64.7041) centre (-13.9242, -65.7053) cw
  line L199 (-14.9253, -65.7054) -> (-14.9253, -73.7149)
  arc A200 (46.3835, -89.7044) -> (45.3823, -88.7032) centre (46.3835, -88.7032) cw
  line L200 (46.3835, -89.7044) -> (54.3931, -89.7044)
  arc A201 (55.3943, -88.7032) -> (54.3931, -89.7044) centre (54.3931, -88.7032) cw
  line L201 (55.3943, -88.7032) -> (55.3943, -80.6936)
  arc A202 (54.3931, -79.6924) -> (55.3943, -80.6936) centre (54.3931, -80.6936) cw
  line L202 (54.3931, -79.6924) -> (46.3835, -79.6924)
  arc A203 (45.3823, -80.6936) -> (46.3835, -79.6924) centre (46.3835, -80.6936) cw
  line L203 (45.3823, -80.6936) -> (45.3823, -88.7032)
  arc A204 (31.3954, -89.7454) -> (30.3942, -88.7443) centre (31.3954, -88.7442) cw
  line L204 (31.3954, -89.7454) -> (39.405, -89.7454)
  arc A205 (40.4061, -88.7443) -> (39.405, -89.7454) centre (39.405, -88.7442) cw
  line L205 (40.4061, -88.7443) -> (40.4061, -80.7347)
  line L206 (39.405, -79.7335) -> (31.3954, -79.7335)
  arc A206 (30.3942, -80.7347) -> (31.3954, -79.7335) centre (31.3954, -80.7347) cw
  line L207 (30.3942, -80.7347) -> (30.3942, -88.7443)
  arc A207 (46.3835, -104.7865) -> (45.3823, -103.7852) centre (46.3835, -103.7853) cw
  line L208 (46.3835, -104.7865) -> (54.3931, -104.7865)
  arc A208 (55.3943, -103.7852) -> (54.3931, -104.7865) centre (54.3931, -103.7853) cw
  line L209 (55.3943, -103.7852) -> (55.3943, -95.7757)
  arc A209 (54.3931, -94.7745) -> (55.3943, -95.7757) centre (54.3931, -95.7757) cw
  line L210 (54.3931, -94.7745) -> (46.3835, -94.7745)
  arc A210 (45.3823, -95.7757) -> (46.3835, -94.7745) centre (46.3835, -95.7757) cw
  line L211 (45.3823, -95.7757) -> (45.3823, -103.7852)
  arc A211 (31.3954, -104.8275) -> (30.3942, -103.8263) centre (31.3954, -103.8263) cw
  line L212 (31.3954, -104.8275) -> (39.405, -104.8275)
  arc A212 (40.4061, -103.8263) -> (39.405, -104.8275) centre (39.405, -103.8263) cw
  line L213 (40.4061, -103.8263) -> (40.4061, -95.8168)
  arc A213 (39.405, -94.8156) -> (40.4061, -95.8168) centre (39.405, -95.8168) cw
  line L214 (39.405, -94.8156) -> (31.3954, -94.8156)
  arc A214 (30.3942, -95.8167) -> (31.3954, -94.8156) centre (31.3954, -95.8168) cw
  line L215 (30.3942, -95.8167) -> (30.3942, -103.8263)
  arc A215 (16.2654, -104.8275) -> (15.2642, -103.8263) centre (16.2654, -103.8263) cw
  line L216 (16.2654, -104.8275) -> (24.275, -104.8275)
  arc A216 (25.2761, -103.8263) -> (24.275, -104.8275) centre (24.275, -103.8263) cw
  line L217 (25.2761, -103.8263) -> (25.2761, -95.8168)
  arc A217 (24.275, -94.8156) -> (25.2761, -95.8168) centre (24.275, -95.8168) cw
  line L218 (24.275, -94.8156) -> (16.2654, -94.8156)
  arc A218 (15.2642, -95.8167) -> (16.2654, -94.8156) centre (16.2654, -95.8168) cw
  line L219 (15.2642, -95.8167) -> (15.2642, -103.8263)
  arc A219 (1.1007, -104.8275) -> (0.0995, -103.8263) centre (1.1007, -103.8263) cw
  line L220 (1.1007, -104.8275) -> (9.1102, -104.8275)
  arc A220 (10.1114, -103.8263) -> (9.1102, -104.8275) centre (9.1102, -103.8263) cw
  line L221 (10.1114, -103.8263) -> (10.1114, -95.8167)
  arc A221 (9.1102, -94.8156) -> (10.1114, -95.8167) centre (9.1102, -95.8168) cw
  line L222 (9.1102, -94.8156) -> (1.1007, -94.8156)
  arc A222 (0.0995, -95.8167) -> (1.1007, -94.8156) centre (1.1007, -95.8168) cw
  line L223 (0.0995, -95.8167) -> (0.0995, -103.8263)
  arc A223 (-13.9242, -104.8275) -> (-14.9253, -103.8263) centre (-13.9242, -103.8263) cw
  line L224 (-13.9242, -104.8275) -> (-5.9146, -104.8275)
  arc A224 (-4.9134, -103.8263) -> (-5.9146, -104.8275) centre (-5.9146, -103.8263) cw
  line L225 (-4.9134, -103.8263) -> (-4.9134, -95.8168)
  arc A225 (-5.9146, -94.8156) -> (-4.9134, -95.8168) centre (-5.9146, -95.8168) cw
  line L226 (-5.9146, -94.8156) -> (-13.9242, -94.8156)
  arc A226 (-14.9253, -95.8168) -> (-13.9242, -94.8156) centre (-13.9242, -95.8168) cw
  line L227 (-14.9253, -95.8168) -> (-14.9253, -103.8263)
  arc A227 (-47.421, -61.7547) -> (-57.6332, -61.7547) centre (-52.5271, -61.7547) cw
  arc A228 (-57.6332, -61.7547) -> (-47.421, -61.7547) centre (-52.5271, -61.7547) cw
  arc A229 (-34.0929, -61.7547) -> (-44.3051, -61.7547) centre (-39.199, -61.7547) cw
  arc A230 (-44.3051, -61.7547) -> (-34.0929, -61.7547) centre (-39.199, -61.7547) cw
  arc A231 (-30.8977, -61.7547) -> (-20.6855, -61.7547) centre (-25.7916, -61.7525) cw
  arc A232 (-20.6855, -61.7547) -> (-30.8977, -61.7547) centre (-25.7916, -61.7569) cw
  arc A233 (-30.8977, -74.5639) -> (-20.6855, -74.5639) centre (-25.7916, -74.5617) cw
  arc A234 (-20.6855, -74.5639) -> (-30.8977, -74.5639) centre (-25.7916, -74.5661) cw
  arc A235 (-34.0929, -74.5639) -> (-44.3051, -74.5639) centre (-39.199, -74.5639) cw
  arc A236 (-44.3051, -74.5639) -> (-34.0929, -74.5639) centre (-39.199, -74.5639) cw
  arc A237 (-47.421, -74.5639) -> (-57.6332, -74.5639) centre (-52.5271, -74.5639) cw
  arc A238 (-57.6332, -74.5639) -> (-47.421, -74.5639) centre (-52.5271, -74.5639) cw
  arc A239 (-30.8977, -87.2934) -> (-20.6855, -87.2934) centre (-25.7916, -87.2912) cw
  arc A240 (-20.6855, -87.2934) -> (-30.8977, -87.2934) centre (-25.7916, -87.2956) cw
  arc A241 (-34.0929, -87.2934) -> (-44.3051, -87.2934) centre (-39.199, -87.2934) cw
  arc A242 (-44.3051, -87.2934) -> (-34.0929, -87.2934) centre (-39.199, -87.2934) cw
  arc A243 (-47.421, -87.2934) -> (-57.6332, -87.2934) centre (-52.5271, -87.2934) cw
  arc A244 (-57.6332, -87.2934) -> (-47.421, -87.2934) centre (-52.5271, -87.2934) cw
  arc A245 (-30.8977, -99.7845) -> (-20.6855, -99.7845) centre (-25.7916, -99.7823) cw
  arc A246 (-20.6855, -99.7845) -> (-30.8977, -99.7845) centre (-25.7916, -99.7867) cw
  arc A247 (-34.0929, -99.7845) -> (-44.3051, -99.7845) centre (-39.199, -99.7845) cw
  arc A248 (-44.3051, -99.7845) -> (-34.0929, -99.7845) centre (-39.199, -99.7845) cw
  arc A249 (-47.421, -99.7845) -> (-57.6332, -99.7845) centre (-52.5271, -99.7845) cw
  arc A250 (-57.6332, -99.7845) -> (-47.421, -99.7845) centre (-52.5271, -99.7845) cw
  circle A251 centre (68.2558, 107.2798) radius 1.3516
  circle A252 centre (-68.1199, 107.225) radius 1.3516
  circle A253 centre (68.2701, 2.396) radius 1.3516
  circle A254 centre (-68.1555, 2.3679) radius 1.3516
  circle A255 centre (68.2335, -93.0365) radius 1.3516
  circle A256 centre (-68.1904, -93) radius 1.3516
  line L228 (51.2525, 93.2445) -> (51.2525, 22.6034)
  spline S0 degree 3 poles (51.2525, 22.6034) (51.2525, 20.8443) (49.8364, 19.4282) (48.0773, 19.4282) knots 0 0 0 0 1 1 1 1
  line L229 (48.0773, 19.4282) -> (-48.0946, 19.4282)
  spline S1 degree 3 poles (-48.0946, 19.4282) (-49.8537, 19.4282) (-51.2697, 20.8443) (-51.2697, 22.6034) knots 0 0 0 0 1 1 1 1
  line L230 (-51.2697, 22.6034) -> (-51.2697, 93.2445)
  spline S2 degree 3 poles (-51.2697, 93.2445) (-51.2697, 95.0036) (-49.8537, 96.4202) (-48.0946, 96.4202) knots 0 0 0 0 1 1 1 1
  line L231 (-48.0946, 96.4202) -> (48.0773, 96.4202)
  spline S3 degree 3 poles (48.0773, 96.4202) (49.8364, 96.4202) (51.2525, 95.0036) (51.2525, 93.2445) knots 0 0 0 0 1 1 1 1
  line L232 (-65.1289, -36.8428) -> (-62.549, -36.8428)
  spline S4 degree 3 poles (-62.549, -36.8428) (-61.8248, -36.8428) (-61.2816, -37.4134) (-61.2816, -38.0717) knots 0 0 0 0 1 1 1 1
  line L233 (-61.2816, -38.0717) -> (-61.2816, -85.3833)
  spline S5 degree 3 poles (-61.2816, -85.3833) (-61.2816, -86.0855) (-61.87, -86.6122) (-62.549, -86.6122) knots 0 0 0 0 1 1 1 1
  line L234 (-62.549, -86.6122) -> (-65.1289, -86.6122)
  spline S6 degree 3 poles (-65.1289, -86.6122) (-65.8531, -86.6122) (-66.3963, -86.0416) (-66.3963, -85.3833) knots 0 0 0 0 1 1 1 1
  line L235 (-66.3963, -85.3833) -> (-66.3963, -38.1156)
  spline S7 degree 3 poles (-66.3963, -38.1156) (-66.3963, -37.4134) (-65.8531, -36.8428) (-65.1289, -36.8428) knots 0 0 0 0 1 1 1 1
  line L236 (61.493, -36.8428) -> (64.073, -36.8428)
  spline S8 degree 3 poles (64.073, -36.8428) (64.7972, -36.8428) (65.3403, -37.4134) (65.3403, -38.0717) knots 0 0 0 0 1 1 1 1
  line L237 (65.3403, -38.0717) -> (65.3403, -85.3833)
  spline S9 degree 3 poles (65.3403, -85.3833) (65.3403, -86.0855) (64.7519, -86.6122) (64.073, -86.6122) knots 0 0 0 0 1 1 1 1
  line L238 (64.073, -86.6122) -> (61.493, -86.6122)
  spline S10 degree 3 poles (61.493, -86.6122) (60.7688, -86.6122) (60.2257, -86.0416) (60.2257, -85.3833) knots 0 0 0 0 1 1 1 1
  line L239 (60.2257, -85.3833) -> (60.2257, -38.1156)
  spline S11 degree 3 poles (60.2257, -38.1156) (60.2257, -37.4134) (60.7688, -36.8428) (61.493, -36.8428) knots 0 0 0 0 1 1 1 1
  spline S12 degree 3 poles (-6.8846, 107.9579) (-6.8846, 109.2471) (-5.8764, 110.3284) (-4.5859, 110.3284) knots 0 0 0 0 1 1 1 1
  line L240 (-4.5859, 110.3284) -> (4.5686, 110.3284)
  spline S13 degree 3 poles (4.5686, 110.3284) (5.8188, 110.3284) (6.8673, 109.2887) (6.8673, 107.9579) knots 0 0 0 0 1 1 1 1
  spline S14 degree 3 poles (6.8673, 107.9579) (6.8673, 106.6687) (5.8591, 105.5874) (4.5686, 105.5874) knots 0 0 0 0 1 1 1 1
  line L241 (4.5686, 105.5874) -> (-4.5859, 105.5874)
  spline S15 degree 3 poles (-4.5859, 105.5874) (-5.836, 105.5874) (-6.8846, 106.6271) (-6.8846, 107.9579) knots 0 0 0 0 1 1 1 1
  spline S16 degree 3 poles (25.2163, 107.9579) (25.2163, 109.2471) (26.2245, 110.3284) (27.515, 110.3284) knots 0 0 0 0 1 1 1 1
  line L242 (27.515, 110.3284) -> (36.6694, 110.3284)
  spline S17 degree 3 poles (36.6694, 110.3284) (37.9196, 110.3284) (38.9681, 109.2887) (38.9681, 107.9579) knots 0 0 0 0 1 1 1 1
  spline S18 degree 3 poles (38.9681, 107.9579) (38.9681, 106.6687) (37.9599, 105.5874) (36.6694, 105.5874) knots 0 0 0 0 1 1 1 1
  line L243 (36.6694, 105.5874) -> (27.515, 105.5874)
  spline S19 degree 3 poles (27.515, 105.5874) (26.2648, 105.5874) (25.2163, 106.6271) (25.2163, 107.9579) knots 0 0 0 0 1 1 1 1
  spline S20 degree 3 poles (9.089, 107.9579) (9.089, 109.2471) (10.0972, 110.3284) (11.3877, 110.3284) knots 0 0 0 0 1 1 1 1
  line L244 (11.3877, 110.3284) -> (20.5421, 110.3284)
  spline S21 degree 3 poles (20.5421, 110.3284) (21.7923, 110.3284) (22.8408, 109.2887) (22.8408, 107.9579) knots 0 0 0 0 1 1 1 1
  spline S22 degree 3 poles (22.8408, 107.9579) (22.8408, 106.6687) (21.8326, 105.5874) (20.5421, 105.5874) knots 0 0 0 0 1 1 1 1
  line L245 (20.5421, 105.5874) -> (11.3877, 105.5874)
  spline S23 degree 3 poles (11.3877, 105.5874) (10.1375, 105.5874) (9.089, 106.6271) (9.089, 107.9579) knots 0 0 0 0 1 1 1 1
  spline S24 degree 3 poles (-38.9854, 107.9579) (-38.9854, 109.2471) (-37.9772, 110.3284) (-36.6867, 110.3284) knots 0 0 0 0 1 1 1 1
  line L246 (-36.6867, 110.3284) -> (-27.5322, 110.3284)
  spline S25 degree 3 poles (-27.5322, 110.3284) (-26.2821, 110.3284) (-25.2335, 109.2887) (-25.2335, 107.9579) knots 0 0 0 0 1 1 1 1
  spline S26 degree 3 poles (-25.2335, 107.9579) (-25.2335, 106.6687) (-26.2417, 105.5874) (-27.5322, 105.5874) knots 0 0 0 0 1 1 1 1
  line L247 (-27.5322, 105.5874) -> (-36.6867, 105.5874)
  spline S27 degree 3 poles (-36.6867, 105.5874) (-37.9368, 105.5874) (-38.9854, 106.6271) (-38.9854, 107.9579) knots 0 0 0 0 1 1 1 1
  spline S28 degree 3 poles (-23.0409, 107.9579) (-23.0409, 109.2472) (-22.0327, 110.3285) (-20.7422, 110.3285) knots 0 0 0 0 1 1 1 1
  line L248 (-20.7422, 110.3285) -> (-11.5878, 110.3285)
  spline S29 degree 3 poles (-11.5878, 110.3285) (-10.3376, 110.3285) (-9.2891, 109.2888) (-9.2891, 107.9579) knots 0 0 0 0 1 1 1 1
  spline S30 degree 3 poles (-9.2891, 107.9579) (-9.2891, 106.6687) (-10.2973, 105.5874) (-11.5878, 105.5874) knots 0 0 0 0 1 1 1 1
  line L249 (-11.5878, 105.5874) -> (-20.7422, 105.5874)
  spline S31 degree 3 poles (-20.7422, 105.5874) (-21.9924, 105.5874) (-23.0409, 106.6271) (-23.0409, 107.9579) knots 0 0 0 0 1 1 1 1
  spline S32 degree 3 poles (72.7563, 111.3749) (72.7483, 112.0136) (72.4689, 112.5845) (72.0273, 112.978) knots 0 0 0 0 1 1 1 1
  spline S33 degree 3 poles (72.0273, 112.978) (71.3865, 113.5491) (69.8626, 113.5296) (68.9848, 113.5296) knots 0 0 0 0 1 1 1 1
  line L250 (68.9848, 113.5296) -> (-68.9979, 113.5296)
  spline S34 degree 3 poles (-68.9979, 113.5296) (-69.8757, 113.5296) (-71.3995, 113.5491) (-72.0404, 112.978) knots 0 0 0 0 1 1 1 1
  spline S35 degree 3 poles (-72.0404, 112.978) (-72.103, 112.9223) (-72.1623, 112.863) (-72.218, 112.8004) knots 0 0 0 0 1 1 1 1
  spline S36 degree 3 poles (-72.218, 112.8004) (-72.7891, 112.1595) (-72.7696, 110.6357) (-72.7696, 109.7579) knots 0 0 0 0 1 1 1 1
  line L251 (-72.7696, 109.7579) -> (-72.7696, 104.5339)
  spline S37 degree 3 poles (-72.7696, 104.5339) (-72.7696, 103.6561) (-72.058, 102.9445) (-71.1802, 102.9445) knots 0 0 0 0 1 1 1 1
  line L252 (-71.1802, 102.9445) -> (-69.9224, 102.9445)
  spline S38 degree 3 poles (-69.9224, 102.9445) (-69.0446, 102.9445) (-67.5869, 102.9725) (-66.7873, 102.6255) knots 0 0 0 0 1 1 1 1
  spline S39 degree 3 poles (-66.7873, 102.6255) (-65.8911, 102.2364) (-65.1731, 101.5185) (-64.7841, 100.6222) knots 0 0 0 0 1 1 1 1
  spline S40 degree 3 poles (-64.7841, 100.6222) (-64.437, 99.8226) (-64.4651, 98.3649) (-64.4651, 97.4871) knots 0 0 0 0 1 1 1 1
  spline S41 degree 3 poles (-64.4651, 97.4871) (-64.4651, 96.8439) (-64.437, 95.5764) (-64.7841, 94.7768) knots 0 0 0 0 1 1 1 1
  spline S42 degree 3 poles (-64.7841, 94.7768) (-65.1731, 93.8805) (-65.8911, 93.1626) (-66.7873, 92.7735) knots 0 0 0 0 1 1 1 1
  spline S43 degree 3 poles (-66.7873, 92.7735) (-67.5869, 92.4265) (-69.0446, 92.4545) (-69.9224, 92.4545) knots 0 0 0 0 1 1 1 1
  line L253 (-69.9224, 92.4545) -> (-71.1802, 92.4545)
  spline S44 degree 3 poles (-71.1802, 92.4545) (-72.058, 92.4545) (-72.7696, 91.743) (-72.7696, 90.8651) knots 0 0 0 0 1 1 1 1
  line L254 (-72.7696, 90.8651) -> (-72.7696, 0.1314)
  spline S45 degree 3 poles (-72.7696, 0.1314) (-72.7696, -0.7464) (-72.058, -1.458) (-71.1802, -1.458) knots 0 0 0 0 1 1 1 1
  line L255 (-71.1802, -1.458) -> (-68.8628, -1.458)
  spline S46 degree 3 poles (-68.8628, -1.458) (-67.985, -1.458) (-66.5273, -1.43) (-65.7277, -1.777) knots 0 0 0 0 1 1 1 1
  spline S47 degree 3 poles (-65.7277, -1.777) (-64.8315, -2.1661) (-64.1135, -2.884) (-63.7245, -3.7803) knots 0 0 0 0 1 1 1 1
  spline S48 degree 3 poles (-63.7245, -3.7803) (-63.3774, -4.5799) (-63.4055, -6.0376) (-63.4055, -6.9154) knots 0 0 0 0 1 1 1 1
  line L256 (-63.4055, -6.9154) -> (-63.4055, -23.5999)
  spline S49 degree 3 poles (-63.4055, -23.5999) (-63.4055, -24.4777) (-63.3775, -25.9354) (-63.7245, -26.735) knots 0 0 0 0 1 1 1 1
  spline S50 degree 3 poles (-63.7245, -26.735) (-64.1135, -27.6313) (-64.8315, -28.3492) (-65.7277, -28.7382) knots 0 0 0 0 1 1 1 1
  spline S51 degree 3 poles (-65.7277, -28.7382) (-66.5273, -29.0853) (-67.985, -29.0573) (-68.8628, -29.0573) knots 0 0 0 0 1 1 1 1
  line L257 (-68.8628, -29.0573) -> (-71.1802, -29.0573)
  spline S52 degree 3 poles (-71.1802, -29.0573) (-72.058, -29.0573) (-72.7696, -29.7689) (-72.7696, -30.6466) knots 0 0 0 0 1 1 1 1
  line L258 (-72.7696, -30.6466) -> (-72.7696, -95.6386)